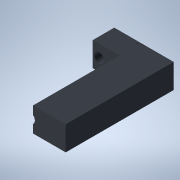
# Autodesk Inventor part: FGR AL-2-PGN-plus-P 160,PGN-plus-P 160-2-AS-P81110452001216049.51650000000000000000Aluminium6.5
Saved by Autodesk Inventor 2021 (Build 250183000, 183)
## iProperties
Created: 2025-07-30
Part Number: FGR AL-2-PGN-plus-P 160,PGN-plus-P 160-2-AS-P81110452001216049.51650000000000000000Aluminium6.5
Material: Generic
Catalog Web Link: www.cadenas.de
Description: FGR-Customizable gripper fingers
Vendor: SCHUNK
Document SubType Name: Modeling
Designer: psAdmin
Manufacturer: SCHUNK
Mass: 613.504 g
Surface Area: 597.818 cm^2
Volume: 613.504 cm^3
Density: 1 g/cm^3
Appearance: PSOLRGB-188-193-204
Category: PARTsolutions
Company: SCHUNK
Title: FGR AL-2-PGN-plus-P 160, 110452002
Author: Cadenas PARTsolutions
Comments: Customizable gripper fingers
PSOL_IDENT_0: {$CADENAS_DATA/23d-libs/schunk/greifsysteme/konfigurationen/system_baukasten/easy_finger/easy_finger
PSOL_IDENT_1: _0421.prj},471 {VTYP=3D},{NB=FGR AL-2-PGN-plus-P 160,PGN-plus-P 160-2-AS-P81110452001216049.51650000
PSOL_IDENT_2: 000000000000Aluminium6.5},{LINA=FGR AL-2-PGN-plus-P 160, 110452002},{NN=FGR},{DATE=13.11.2024 09:26:
PSOL_IDENT_3: 27},{GEOMDATE=20.06.2024 14:57:51},{VERSION=},{LINEID=10},{WBVAR=BR,BGVR,ASIS,SPANNKONT,CNSMAT,HUB,R
PSOL_IDENT_4: H,X,Y,Z,ABK,DWS,GFL,GFT,PP,PW,RA,EFO,FASE1,FL1,FASE2,FL2,FASE3,FW3,FL3,FASE4,FW4,FL4,WAERMEBE,BM},{W
PSOL_IDENT_5: BNUMERIC=HUB,RH,X,Y,Z,ABK,DWS,GFL,GFT,PP,PW,RA,EFO,FL1,FL2,FASE3,FW3,FL3,FW4,FL4,BM}  {NB=FGR AL-2-P
PSOL_IDENT_6: GN-plus-P 160,PGN-plus-P 160-2-AS-P81110452001216049.51650000000000000000Aluminium6.5},{LINA=FGR AL-
PSOL_IDENT_7: 2-PGN-plus-P 160, 110452002},{KT=DUMMY},{START=Geometriemodell 2},{VERSION=1},{VER=V1},{MATN=3786171
PSOL_IDENT_8: 200_fgr_gl_ia_v1},{XMLMATN=material|},{XMLMAT=AlZn55MgCu_EN-AW-7075_34365},{TYP=FGR AL-2-PGN-plus-P
PSOL_IDENT_9: 160},{TYPX=PGN-plus-P 160},{TYPXX=PGN-plus-P 160},{TYPXMAT=AL},{BR=PGN-plus-P},{BG=160.0},{BGVR=PGN-
PSOL_IDENT_10: plus-P 160-2-AS-P},{BGVRX='PGN-plus-P 40','PGN-plus-P 40','PGN-plus-P 40-SD','PGN-plus-P 40-SD','PGN
PSOL_IDENT_11: -plus-P 40-K','PGN-plus-P 40-K','PGN-plus-P 40-V','PGN-plus-P 40-V','PGN-plus-P 40-P','PGN-plus-P 40
PSOL_IDENT_12: -P','PGN-plus-P 40-AS','PGN-plus-P 40-AS','PGN-plus-P 40-AS-SD','PGN-plus-P 40-AS-SD','PGN-plus-P 40
PSOL_IDENT_13: -AS-K','PGN-plus-P 40-AS-K','PGN-plus-P 40-AS-V','PGN-plus-P 40-AS-V','PGN-plus-P 40-AS-P','PGN-plus
PSOL_IDENT_14: -P 40-AS-P','PGN-plus-P 40-IS','PGN-plus-P 40-IS','PGN-plus-P 40-IS-SD','PGN-plus-P 40-IS-SD','PGN-p
PSOL_IDENT_15: lus-P 40-IS-K','PGN-plus-P 40-IS-K','PGN-plus-P 40-IS-V','PGN-plus-P 40-IS-V','PGN-plus-P 50-1','PGN
PSOL_IDENT_16: -plus-P 50-1','PGN-plus-P 50-1-SD','PGN-plus-P 50-1-SD','PGN-plus-P 50-1-K','PGN-plus-P 50-1-K','PGN
PSOL_IDENT_17: -plus-P 50-1-V','PGN-plus-P 50-1-V','PGN-plus-P 50-1-P','PGN-plus-P 50-1-P','PGN-plus-P 50-2','PGN-p
PSOL_IDENT_18: lus-P 50-2','PGN-plus-P 50-2-SD','PGN-plus-P 50-2-SD','PGN-plus-P 50-2-K','PGN-plus-P 50-2-K','PGN-p
PSOL_IDENT_19: lus-P 50-2-V','PGN-plus-P 50-2-V','PGN-plus-P 50-2-P','PGN-plus-P 50-2-P','PGN-plus-P 50-1-AS','PGN-
PSOL_IDENT_20: plus-P 50-1-AS','PGN-plus-P 50-1-AS-SD','PGN-plus-P 50-1-AS-SD','PGN-plus-P 50-1-AS-K','PGN-plus-P 5
PSOL_IDENT_21: 0-1-AS-K','PGN-plus-P 50-1-AS-V','PGN-plus-P 50-1-AS-V','PGN-plus-P 50-1-AS-P','PGN-plus-P 50-1-AS-P'
PSOL_IDENT_22: ,'PGN-plus-P 50-2-AS','PGN-plus-P 50-2-AS','PGN-plus-P 50-2-AS-SD','PGN-plus-P 50-2-AS-SD','PGN-plus
PSOL_IDENT_23: -P 50-2-AS-K','PGN-plus-P 50-2-AS-K','PGN-plus-P 50-2-AS-V','PGN-plus-P 50-2-AS-V','PGN-plus-P 50-2-
PSOL_IDENT_24: AS-P','PGN-plus-P 50-2-AS-P','PGN-plus-P 50-1-IS','PGN-plus-P 50-1-IS','PGN-plus-P 50-1-IS-SD','PGN-
PSOL_IDENT_25: plus-P 50-1-IS-SD','PGN-plus-P 50-1-IS-K','PGN-plus-P 50-1-IS-K','PGN-plus-P 50-1-IS-V','PGN-plus-P
PSOL_IDENT_26: 50-1-IS-V','PGN-plus-P 50-2-IS','PGN-plus-P 50-2-IS','PGN-plus-P 50-2-IS-SD','PGN-plus-P 50-2-IS-SD'
PSOL_IDENT_27: ,'PGN-plus-P 50-2-IS-K','PGN-plus-P 50-2-IS-K','PGN-plus-P 50-2-IS-V','PGN-plus-P 50-2-IS-V','PGN-pl
PSOL_IDENT_28: us-P 64-1','PGN-plus-P 64-1','PGN-plus-P 64-1-SD','PGN-plus-P 64-1-SD','PGN-plus-P 64-1-K','PGN-plus
PSOL_IDENT_29: -P 64-1-K','PGN-plus-P 64-1-V','PGN-plus-P 64-1-V','PGN-plus-P 64-1-P','PGN-plus-P 64-1-P','PGN-plus
PSOL_IDENT_30: -P 64-2','PGN-plus-P 64-2','PGN-plus-P 64-2-SD','PGN-plus-P 64-2-SD','PGN-plus-P 64-2-K','PGN-plus-P
PSOL_IDENT_31: 64-2-K','PGN-plus-P 64-2-V','PGN-plus-P 64-2-V','PGN-plus-P 64-2-P','PGN-plus-P 64-2-P','PGN-plus-P
PSOL_IDENT_32: 64-1-AS','PGN-plus-P 64-1-AS','PGN-plus-P 64-1-AS-SD','PGN-plus-P 64-1-AS-SD','PGN-plus-P 64-1-AS-K'
PSOL_IDENT_33: ,'PGN-plus-P 64-1-AS-K','PGN-plus-P 64-1-AS-V','PGN-plus-P 64-1-AS-V','PGN-plus-P 64-1-AS-P','PGN-pl
PSOL_IDENT_34: us-P 64-1-AS-P','PGN-plus-P 64-2-AS','PGN-plus-P 64-2-AS','PGN-plus-P 64-1-IS','PGN-plus-P 64-1-IS','
PSOL_IDENT_35: PGN-plus-P 64-1-IS-SD','PGN-plus-P 64-1-IS-SD','PGN-plus-P 64-1-IS-K','PGN-plus-P 64-1-IS-K','PGN-pl
PSOL_IDENT_36: us-P 64-1-IS-V','PGN-plus-P 64-1-IS-V','PGN-plus-P 64-2-IS','PGN-plus-P 64-2-IS','PGN-plus-P 64-2-IS
PSOL_IDENT_37: -SD','PGN-plus-P 64-2-IS-SD','PGN-plus-P 64-2-IS-K','PGN-plus-P 64-2-IS-K','PGN-plus-P 64-2-V','PGN-
PSOL_IDENT_38: plus-P 64-2-V','PGN-plus-P 80-1','PGN-plus-P 80-1','PGN-plus-P 80-1-SD','PGN-plus-P 80-1-SD','PGN-pl
PSOL_IDENT_39: us-P 80-1-K','PGN-plus-P 80-1-K','PGN-plus-P 80-1-V','PGN-plus-P 80-1-V','PGN-plus-P 80-1-P','PGN-pl
PSOL_IDENT_40: us-P 80-1-P','PGN-plus-P 80-2','PGN-plus-P 80-2','PGN-plus-P 80-2-SD','PGN-plus-P 80-2-SD','PGN-plus
PSOL_IDENT_41: -P 80-2-K','PGN-plus-P 80-2-K','PGN-plus-P 80-2-V','PGN-plus-P 80-2-V','PGN-plus-P 80-2-P','PGN-plus
PSOL_IDENT_42: -P 80-2-P','PGN-plus-P 80-1-AS','PGN-plus-P 80-1-AS','PGN-plus-P 80-1-AS-SD','PGN-plus-P 80-1-AS-SD'
PSOL_IDENT_43: ,'PGN-plus-P 80-1-AS-K','PGN-plus-P 80-1-AS-K','PGN-plus-P 80-1-AS-V','PGN-plus-P 80-1-AS-V','PGN-pl
PSOL_IDENT_44: us-P 80-1-AS-P','PGN-plus-P 80-1-AS-P','PGN-plus-P 80-2-AS','PGN-plus-P 80-2-AS','PGN-plus-P 80-2-AS
PSOL_IDENT_45: -SD', 'PGN-plus-P 80-2-AS-SD','PGN-plus-P 80-2-AS-K','PGN-plus-P 80-2-AS-K','PGN-plus-P 80-2-AS-V','
PSOL_IDENT_46: PGN-plus-P 80-2-AS-V','PGN-plus-P 80-2-AS-P','PGN-plus-P 80-2-AS-P','PGN-plus-P 80-1-IS','PGN-plus-P
PSOL_IDENT_47: 80-1-IS','PGN-plus-P 80-1-IS-SD','PGN-plus-P 80-1-IS-SD','PGN-plus-P 80-1-IS-K','PGN-plus-P 80-1-IS
PSOL_IDENT_48: -K','PGN-plus-P 80-1-IS-V','PGN-plus-P 80-1-IS-V','PGN-plus-P 80-2-IS','PGN-plus-P 80-2-IS','PGN-plu
PSOL_IDENT_49: s-P 80-2-IS-SD','PGN-plus-P 80-2-IS-SD','PGN-plus-P 80-2-IS-K','PGN-plus-P 80-2-IS-K','PGN-plus-P 80
PSOL_IDENT_50: -2-IS-V','PGN-plus-P 80-2-IS-V','PGN-plus-P 100-1','PGN-plus-P 100-1','PGN-plus-P 100-1-SD','PGN-plu
PSOL_IDENT_51: s-P 100-1-SD','PGN-plus-P 100-1-K','PGN-plus-P 100-1-K','PGN-plus-P 100-1-V','PGN-plus-P 100-1-V','P
PSOL_IDENT_52: GN-plus-P 100-1-P','PGN-plus-P 100-1-P','PGN-plus-P 100-2','PGN-plus-P 100-2','PGN-plus-P 100-2-SD','
PSOL_IDENT_53: PGN-plus-P 100-2-SD','PGN-plus-P 100-2-K','PGN-plus-P 100-2-K','PGN-plus-P 100-2-V','PGN-plus-P 100-
PSOL_IDENT_54: 2-V','PGN-plus-P 100-2-P','PGN-plus-P 100-2-P','PGN-plus-P 100-1-AS','PGN-plus-P 100-1-AS','PGN-plus
PSOL_IDENT_55: -P 100-1-AS-SD','PGN-plus-P 100-1-AS-SD','PGN-plus-P 100-1-AS-K','PGN-plus-P 100-1-AS-K','PGN-plus-P
PSOL_IDENT_56: 100-1-AS-V','PGN-plus-P 100-1-AS-V','PGN-plus-P 100-1-AS-P','PGN-plus-P 100-1-AS-P','PGN-plus-P 100
PSOL_IDENT_57: -2-AS','PGN-plus-P 100-2-AS','PGN-plus-P 100-2-AS-SD','PGN-plus-P 100-2-AS-SD','PGN-plus-P 100-2-AS-
PSOL_IDENT_58: K','PGN-plus-P 100-2-AS-K','PGN-plus-P 100-2-AS-V','PGN-plus-P 100-2-AS-V','PGN-plus-P 100-2-AS-P','
PSOL_IDENT_59: PGN-plus-P 100-2-AS-P','PGN-plus-P 100-1-IS','PGN-plus-P 100-1-IS','PGN-plus-P 100-1-IS-SD','PGN-plu
PSOL_IDENT_60: s-P 100-1-IS-SD','PGN-plus-P 100-1-IS-K','PGN-plus-P 100-1-IS-K','PGN-plus-P 100-1-IS-V','PGN-plus-P
PSOL_IDENT_61: 100-1-IS-V','PGN-plus-P 100-2-IS','PGN-plus-P 100-2-IS','PGN-plus-P 100-2-IS-SD','PGN-plus-P 100-2-
PSOL_IDENT_62: IS-SD','PGN-plus-P 100-2-IS-K','PGN-plus-P 100-2-IS-K','PGN-plus-P 100-2-IS-V','PGN-plus-P 100-2-IS-
PSOL_IDENT_63: V','PGN-plus-P 125-1','PGN-plus-P 125-1','PGN-plus-P 125-1-SD','PGN-plus-P 125-1-SD','PGN-plus-P 125
PSOL_IDENT_64: -1-K','PGN-plus-P 125-1-K','PGN-plus-P 125-1-V','PGN-plus-P 125-1-V','PGN-plus-P 125-1-P','PGN-plus-
PSOL_IDENT_65: P 125-1-P','PGN-plus-P 125-2','PGN-plus-P 125-2','PGN-plus-P 125-2-SD','PGN-plus-P 125-2-SD','PGN-pl
PSOL_IDENT_66: us-P 125-2-K','PGN-plus-P 125-2-K','PGN-plus-P 125-2-V','PGN-plus-P 125-2-V','PGN-plus-P 125-2-P','P
PSOL_IDENT_67: GN-plus-P 125-2-P','PGN-plus-P 125-1-AS','PGN-plus-P 125-1-AS','PGN-plus-P 125-1-AS-SD','PGN-plus-P
PSOL_IDENT_68: 125-1-AS-SD','PGN-plus-P 125-1-AS-K','PGN-plus-P 125-1-AS-K','PGN-plus-P 125-1-AS-V','PGN-plus-P 125
PSOL_IDENT_69: -1-AS-V','PGN-plus-P 125-1-AS-P','PGN-plus-P 125-1-AS-P','PGN-plus-P 125-2-AS','PGN-plus-P 125-2-AS'
PSOL_IDENT_70: ,'PGN-plus-P 125-2-AS-SD','PGN-plus-P 125-2-AS-SD','PGN-plus-P 125-2-AS-K','PGN-plus-P 125-2-AS-K','
PSOL_IDENT_71: PGN-plus-P 125-2-AS-V','PGN-plus-P 125-2-AS-V','PGN-plus-P 125-2-AS-P','PGN-plus-P 125-2-AS-P','PGN-
PSOL_IDENT_72: plus-P 125-1-IS','PGN-plus-P 125-1-IS','PGN-plus-P 125-1-IS-SD','PGN-plus-P 125-1-IS-SD','PGN-plus-P
PSOL_IDENT_73: 125-1-IS-K','PGN-plus-P 125-1-IS-K','PGN-plus-P 125-1-IS-V','PGN-plus-P 125-1-IS-V','PGN-plus-P 125
PSOL_IDENT_74: -2-IS','PGN-plus-P 125-2-IS','PGN-plus-P 125-2-IS-SD','PGN-plus-P 125-2-IS-SD','PGN-plus-P 125-2-IS-
PSOL_IDENT_75: K','PGN-plus-P 125-2-IS-K','PGN-plus-P 125-2-IS-V','PGN-plus-P 125-2-IS-V','PGN-plus-P 160-1','PGN-p
PSOL_IDENT_76: lus-P 160-1','PGN-plus-P 160-1-SD','PGN-plus-P 160-1-SD','PGN-plus-P 160-1-K','PGN-plus-P 160-1-K','
PSOL_IDENT_77: PGN-plus-P 160-1-V','PGN-plus-P 160-1-V','PGN-plus-P 160-1-P','PGN-plus-P 160-1-P','PGN-plus-P 160-2'
PSOL_IDENT_78: ,'PGN-plus-P 160-2','PGN-plus-P 160-2-SD','PGN-plus-P 160-2-SD','PGN-plus-P 160-2-K','PGN-plus-P 160
PSOL_IDENT_79: -2-K','PGN-plus-P 160-2-V','PGN-plus-P 160-2-V','PGN-plus-P 160-2-P','PGN-plus-P 160-2-P','PGN-plus-
PSOL_IDENT_80: P 160-1-AS','PGN-plus-P 160-1-AS','PGN-plus-P 160-1-AS-SD','PGN-plus-P 160-1-AS-SD','PGN-plus-P 160-
PSOL_IDENT_81: 1-AS-K','PGN-plus-P 160-1-AS-K','PGN-plus-P 160-1-AS-V','PGN-plus-P 160-1-AS-V','PGN-plus-P 160-1-AS
PSOL_IDENT_82: -P','PGN-plus-P 160-1-AS-P','PGN-plus-P 160-2-AS','PGN-plus-P 160-2-AS','PGN-plus-P 160-2-AS-SD','PG
PSOL_IDENT_83: N-plus-P 160-2-AS-SD','PGN-plus-P 160-2-AS-K','PGN-plus-P 160-2-AS-K','PGN-plus-P 160-2-AS-V','PGN-p
PSOL_IDENT_84: lus-P 160-2-AS-V','PGN-plus-P 160-2-AS-P','PGN-plus-P 160-2-AS-P','PGN-plus-P 160-1-IS','PGN-plus-P
PSOL_IDENT_85: 160-1-IS','PGN-plus-P 160-1-IS-SD','PGN-plus-P 160-1-IS-SD','PGN-plus-P 160-1-IS-K','PGN-plus-P 160-
PSOL_IDENT_86: 1-IS-K','PGN-plus-P 160-1-IS-V','PGN-plus-P 160-1-IS-V','PGN-plus-P 160-2-IS','PGN-plus-P 160-2-IS','
PSOL_IDENT_87: PGN-plus-P 160-2-IS-SD','PGN-plus-P 160-2-IS-SD','PGN-plus-P 160-2-IS-K','PGN-plus-P 160-2-IS-K','PG
PSOL_IDENT_88: N-plus-P 160-2-IS-V','PGN-plus-P 160-2-IS-V','PGN-plus-P 200-1','PGN-plus-P 200-1','PGN-plus-P 200-1
PSOL_IDENT_89: -SD','PGN-plus-P 200-1-SD','PGN-plus-P 200-1-K','PGN-plus-P 200-1-K','PGN-plus-P 200-1-V','PGN-plus-
PSOL_IDENT_90: P 200-1-V','PGN-plus-P 200-1-P','PGN-plus-P 200-1-P','PGN-plus-P 200-2','PGN-plus-P 200-2','PGN-plus
PSOL_IDENT_91: -P 200-2-SD','PGN-plus-P 200-2-SD','PGN-plus-P 200-2-K','PGN-plus-P 200-2-K','PGN-plus-P 200-2-V','P
PSOL_IDENT_92: GN-plus-P 200-2-V','PGN-plus-P 200-2-P','PGN-plus-P 200-2-P','PGN-plus-P 200-1-AS','PGN-plus-P 200-1
PSOL_IDENT_93: -AS','PGN-plus-P 200-1-AS-SD','PGN-plus-P 200-1-AS-SD','PGN-plus-P 200-1-AS-K','PGN-plus-P 200-1-AS-
PSOL_IDENT_94: K','PGN-plus-P 200-1-AS-V','PGN-plus-P 200-1-AS-V','PGN-plus-P 200-1-AS-P','PGN-plus-P 200-1-AS-P','
PSOL_IDENT_95: PGN-plus-P 200-2-AS','PGN-plus-P 200-2-AS','PGN-plus-P 200-2-AS-SD','PGN-plus-P 200-2-AS-SD','PGN-pl
PSOL_IDENT_96: us-P 200-2-AS-K','PGN-plus-P 200-2-AS-K','PGN-plus-P 200-2-AS-V','PGN-plus-P 200-2-AS-V','PGN-plus-P
PSOL_IDENT_97: 200-2-AS-P','PGN-plus-P 200-2-AS-P','PGN-plus-P 200-1-IS','PGN-plus-P 200-1-IS','PGN-plus-P 200-1-I
PSOL_IDENT_98: S-SD','PGN-plus-P 200-1-IS-SD','PGN-plus-P 200-1-IS-K','PGN-plus-P 200-1-IS-K','PGN-plus-P 200-1-IS-
PSOL_IDENT_99: V','PGN-plus-P 200-1-IS-V','PGN-plus-P 200-2-IS','PGN-plus-P 200-2-IS','PGN-plus-P 200-2-IS-SD','PGN
PSOL_IDENT_100: -plus-P 200-2-IS-SD','PGN-plus-P 200-2-IS-K','PGN-plus-P 200-2-IS-K','PGN-plus-P 200-2-IS-V','PGN-pl
PSOL_IDENT_101: us-P 200-2-IS-V','PGN-plus-P 240-1','PGN-plus-P 240-1','PGN-plus-P 240-1-SD','PGN-plus-P 240-1-SD','
PSOL_IDENT_102: PGN-plus-P 240-1-K','PGN-plus-P 240-1-K','PGN-plus-P 240-1-V','PGN-plus-P 240-1-V','PGN-plus-P 240-1
PSOL_IDENT_103: -P','PGN-plus-P 240-1-P','PGN-plus-P 240-2','PGN-plus-P 240-2','PGN-plus-P 240-2-SD','PGN-plus-P 240
PSOL_IDENT_104: -2-SD','PGN-plus-P 240-2-K','PGN-plus-P 240-2-K','PGN-plus-P 240-2-V','PGN-plus-P 240-2-V','PGN-plus
PSOL_IDENT_105: -P 240-2-P','PGN-plus-P 240-2-P', 'PGN-plus-P 240-1-AS','PGN-plus-P 240-1-AS','PGN-plus-P 240-1-AS-S
PSOL_IDENT_106: D','PGN-plus-P 240-1-AS-SD','PGN-plus-P 240-1-AS-K','PGN-plus-P 240-1-AS-K','PGN-plus-P 240-1-AS-V','
PSOL_IDENT_107: PGN-plus-P 240-1-AS-V','PGN-plus-P 240-1-AS-P','PGN-plus-P 240-1-AS-P', 'PGN-plus-P 240-2-AS','PGN-p
PSOL_IDENT_108: lus-P 240-2-AS','PGN-plus-P 240-2-AS-SD','PGN-plus-P 240-2-AS-SD','PGN-plus-P 240-2-AS-K','PGN-plus-
PSOL_IDENT_109: P 240-2-AS-K','PGN-plus-P 240-2-AS-V','PGN-plus-P 240-2-AS-V','PGN-plus-P 240-2-AS-P','PGN-plus-P 24
PSOL_IDENT_110: 0-2-AS-P', 'PGN-plus-P 240-1-IS','PGN-plus-P 240-1-IS','PGN-plus-P 240-1-IS-SD','PGN-plus-P 240-1-IS
PSOL_IDENT_111: -SD','PGN-plus-P 240-1-IS-K','PGN-plus-P 240-1-IS-K','PGN-plus-P 240-1-IS-V','PGN-plus-P 240-1-IS-V'
PSOL_IDENT_112: , 'PGN-plus-P 240-2-IS','PGN-plus-P 240-2-IS','PGN-plus-P 240-2-IS-SD','PGN-plus-P 240-2-IS-SD','PGN
PSOL_IDENT_113: -plus-P 240-2-IS-K','PGN-plus-P 240-2-IS-K','PGN-plus-P 240-2-IS-V','PGN-plus-P 240-2-IS-V','PGN-plu
PSOL_IDENT_114: s-P 300-1','PGN-plus-P 300-1','PGN-plus-P 300-1-SD','PGN-plus-P 300-1-SD','PGN-plus-P 300-1-K','PGN-
PSOL_IDENT_115: plus-P 300-1-K','PGN-plus-P 300-1-V','PGN-plus-P 300-1-V','PGN-plus-P 300-1-P','PGN-plus-P 300-1-P','
PSOL_IDENT_116: PGN-plus-P 300-2','PGN-plus-P 300-2','PGN-plus-P 300-2-SD','PGN-plus-P 300-2-SD','PGN-plus-P 300-2-K'
PSOL_IDENT_117: ,'PGN-plus-P 300-2-K','PGN-plus-P 300-2-V','PGN-plus-P 300-2-V','PGN-plus-P 300-2-P','PGN-plus-P 300
PSOL_IDENT_118: -2-P', 'PGN-plus-P 300-1-AS','PGN-plus-P 300-1-AS','PGN-plus-P 300-1-AS-SD','PGN-plus-P 300-1-AS-SD'
PSOL_IDENT_119: ,'PGN-plus-P 300-1-AS-K','PGN-plus-P 300-1-AS-K','PGN-plus-P 300-1-AS-V','PGN-plus-P 300-1-AS-V','PG
PSOL_IDENT_120: N-plus-P 300-1-AS-P','PGN-plus-P 300-1-AS-P', 'PGN-plus-P 300-2-AS','PGN-plus-P 300-2-AS','PGN-plus-
PSOL_IDENT_121: P 300-2-AS-SD','PGN-plus-P 300-2-AS-SD','PGN-plus-P 300-2-AS-K','PGN-plus-P 300-2-AS-K','PGN-plus-P
PSOL_IDENT_122: 300-2-AS-V','PGN-plus-P 300-2-AS-V','PGN-plus-P 300-2-AS-P','PGN-plus-P 300-2-AS-P', 'PGN-plus-P 300
PSOL_IDENT_123: -1-IS','PGN-plus-P 300-1-IS','PGN-plus-P 300-1-IS-SD','PGN-plus-P 300-1-IS-SD','PGN-plus-P 300-1-IS-
PSOL_IDENT_124: K','PGN-plus-P 300-1-IS-K','PGN-plus-P 300-1-IS-V','PGN-plus-P 300-1-IS-V', 'PGN-plus-P 300-2-IS','P
PSOL_IDENT_125: GN-plus-P 300-2-IS','PGN-plus-P 300-2-IS-SD','PGN-plus-P 300-2-IS-SD','PGN-plus-P 300-2-IS-K','PGN-p
PSOL_IDENT_126: lus-P 300-2-IS-K','PGN-plus-P 300-2-IS-V','PGN-plus-P 300-2-IS-V','PGN-plus-P 380-1','PGN-plus-P 380
PSOL_IDENT_127: -1','PGN-plus-P 380-1-SD','PGN-plus-P 380-1-SD','PGN-plus-P 380-1-K','PGN-plus-P 380-1-K','PGN-plus-
PSOL_IDENT_128: P 380-1-V','PGN-plus-P 380-1-V','PGN-plus-P 380-1-P','PGN-plus-P 380-1-P','PGN-plus-P 380-2','PGN-pl
PSOL_IDENT_129: us-P 380-2','PGN-plus-P 380-2-SD','PGN-plus-P 380-2-SD','PGN-plus-P 380-2-K','PGN-plus-P 380-2-K','P
PSOL_IDENT_130: GN-plus-P 380-2-V','PGN-plus-P 380-2-V','PGN-plus-P 380-2-P','PGN-plus-P 380-2-P', 'PGN-plus-P 380-1
PSOL_IDENT_131: -AS','PGN-plus-P 380-1-AS','PGN-plus-P 380-1-AS-SD','PGN-plus-P 380-1-AS-SD','PGN-plus-P 380-1-AS-K'
PSOL_IDENT_132: ,'PGN-plus-P 380-1-AS-K','PGN-plus-P 380-1-AS-V','PGN-plus-P 380-1-AS-V','PGN-plus-P 380-1-AS-P','PG
PSOL_IDENT_133: N-plus-P 380-1-AS-P', 'PGN-plus-P 380-2-AS','PGN-plus-P 380-2-AS','PGN-plus-P 380-2-AS-SD','PGN-plus
PSOL_IDENT_134: -P 380-2-AS-SD','PGN-plus-P 380-2-AS-K','PGN-plus-P 380-2-AS-K','PGN-plus-P 380-2-AS-V','PGN-plus-P
PSOL_IDENT_135: 380-2-AS-V','PGN-plus-P 380-2-AS-P','PGN-plus-P 380-2-AS-P', 'PGN-plus-P 380-1-IS','PGN-plus-P 380-1
PSOL_IDENT_136: -IS','PGN-plus-P 380-1-IS-SD','PGN-plus-P 380-1-IS-SD','PGN-plus-P 380-1-IS-K','PGN-plus-P 380-1-IS-
PSOL_IDENT_137: K','PGN-plus-P 380-1-IS-V','PGN-plus-P 380-1-IS-V', 'PGN-plus-P 380-2-IS','PGN-plus-P 380-2-IS','PGN
PSOL_IDENT_138: -plus-P 380-2-IS-SD','PGN-plus-P 380-2-IS-SD','PGN-plus-P 380-2-IS-K','PGN-plus-P 380-2-IS-K','PGN-p
PSOL_IDENT_139: lus-P 380-2-IS-V','PGN-plus-P 380-2-IS-V'},{IDNR=1317660},{ASIS=1},{ASISX=<'1','Außengreifen','ausse
PSOL_IDENT_140: ngreifen.png'>,'2','Innnengreifen','innengreifen.png'},{ASISXX=AS},{SPANNKONT=2},{SPANNKONTX='1', 'G
PSOL_IDENT_141: erader Greiferfinger', 'startmodell_1.png', '2' , 'Greiferfinger mit nach innen abgesetzter Greifflä
PSOL_IDENT_142: che', 'startmodell_2.png', '3' , 'Greiferfinger mit nach außen abgesetzter Greiffläche', 'startmodel
PSOL_IDENT_143: l_3.png', '4' , 'Greiferfinger mit nach innen abgesetzter und abgerundeter Greiffläche', 'startmodel
PSOL_IDENT_144: l_4.png', '5' , 'Greiferfinger mit nach außen abgesetzter und abgerundeter Greiffläche', 'startmodel
PSOL_IDENT_145: l_5.png', '6' , 'Greiferfinger mit nach innen abgesetzter Greiffläche und vertikalem Prisma', 'start
PSOL_IDENT_146: modell_6.png','8' , 'Greiferfinger mit horizontalem Prisma', 'startmodell_8.png'},{CNSMAT=Aluminium}
PSOL_IDENT_147: ,{HUB=8.0},{HMAX=8.0},{RH=6.5},{HMAXX=8.0},{RHB=2.0},{AB=32.0},{GFM=38.50},{GFMAS=38.50},{GFMIS=70.5
PSOL_IDENT_148: 0},{X=110.0},{XMIN=56.0},{XMAX=113.0},{XTEST=[56:113/0.1]},{MAXX=113.0},{Y=45.0},{YMIN=27.0},{YMAX=6
PSOL_IDENT_149: 0.0},{MAXY=60.0},{Z=200.0},{ZMIN=32.0},{ZMAX=200.0},{ZMAXX=100.0},{MAXZ=200.0},{ABK=12.00},{ABKMIN=1
PSOL_IDENT_150: 2.00},{ABKMAX=37.50},{DWS=165.0},{DWSX=[68:222]},{DWSMIN=68.000},{DWSMAX=222.000},{DWSMAXX=111.0},{D
PSOL_IDENT_151: WSXX=1.000},{DWSZ=1.000},{DWS1V=70.0},{DWS1H=110.0},{DWS2V=134.0},{DWS2H=174.0},{DWSK=134.0},{GWI=1.
PSOL_IDENT_152: 0},{GFL=160.0},{GFLX=[1:169.4]},{GFLMIN=1.00},{GFLMAX=169.40},{GFT=49.50},{GFTX=[49.5:49.5/0.1]},{GF
PSOL_IDENT_153: TMIN=49.50},{GFTMINTH=-217577236067824.12},{GFTMAX=49.50},{GFT1V=2.00},{GFT1H=22.00},{GFT2V=34.00},{
PSOL_IDENT_154: GFT2H=54.00},{SKS=10.6},{PP=0.0},{PPX=[0]},{PPMIN=0.0},{PPMAX=0.0},{PUK=0.00},{PUKZ=88.50},{PUKX=0.0
PSOL_IDENT_155: 0},{PW=0.0},{PWX=[0]},{PWMIN=120},{PWMAX=120},{PWTH=120.0},{PWTHX=180.000},{ALPHA=0.000},{RA=0.0},{R
PSOL_IDENT_156: AX=[0]},{RAMIN=1},{RAMAX=44},{EFO=0.0},{EFOX=[0]},{EFOMAX=0.10},{FASE1=0},{FASE1X='0','ohne Fase 1','
PSOL_IDENT_157: kein_bild.png','1','mit Fase 1','fase_1.png'},{FW1=0.0},{FL1=0.0},{FL1MIN=0.0},{FL1MAX=0.0},{FASE2=0
PSOL_IDENT_158: },{FASE2X='0','ohne Fase 2','kein_bild.png','1','mit Fase 2','fase_2.png'},{FW2=0.0},{FL2=0.0},{FL2M
PSOL_IDENT_159: IN=0.0},{FL2MAX=0.00},{FASE3=0},{FW3=0.0},{FW3MIN=0.0},{FW3MAX=0.0},{FL3=0.0},{FL3MIN=0.0},{FL3MAX=0
PSOL_IDENT_160: .00},{FASE4=0},{FASE4X='0','ohne Fase 4','kein_bild.png','1','mit Fase 4','fase_4_glatt.png'},{FW4=0
PSOL_IDENT_161: .0},{FW4MIN=0.0},{FW4MAX=0.0},{FL4=0.0},{FL4MIN=0.0},{FL4MAX=0.00},{ROHX=2.683},{ROH=1.457},{ZULFM=3
PSOL_IDENT_162: .800},{VALFM=true},{VOL=537767.200},{VFASE1=0.00},{VFASE2=0.00},{VFASE3=0.00},{VFASE4=0.00},{GFTXX=2
PSOL_IDENT_163: .00},{STX1=20.00},{STX2=20.00},{EST=17.0},{ZD=14.0},{ZT=4.0},{DB=11.0},{SD=18.0},{ST=20.0},{RI=8.2},
PSOL_IDENT_164: {L=6.5},{LX=-31},{L1=1.000},{L1X=-0.000},{L2=1.000},{LA=82.500},{GANS=M10},{PBO=11.0},{DPB=11.00},{R
PSOL_IDENT_165: PO=3},{AQB=2.75},{SCHT=0.75},{SCHL=17.40},{SCHH=6.40},{SCHP=5.00},{TYPALU=3.00},{SCHGD=10.0},{SCHGL=
PSOL_IDENT_166: 35.0},{LZ=5 Werktage},{VK=272.00},{VKB=226.11},{VKZ=33.92},{VKX=11.31},{VKP=0.00},{ZX=200.00},{ZXX=1
PSOL_IDENT_167: 00.00},{XX=113.00},{XXX=56.50},{SPERR=0.00},{WC=3786171200_fgr_gl_ia_v1.prt},{MN=3786171200_FGR_GL_I
PSOL_IDENT_168: A_V1},{XMLX=dim|15},{XMLY=dim|14},{XMLZ=dim|13},{XMLAB=dim|35},{XMLABK=dim|71},{XMLGFL=dim|70},{XMLG
PSOL_IDENT_169: FT=dim|68},{XMLFL1=dim|188},{XMLFL2=dim|151},{XMLFL3=dim|272},{XMLFW3=dim|274},{XMLFL4=dim|212},{XML
PSOL_IDENT_170: FW4=dim|211},{XMLRA=},{XMLRI=},{XMLPW=},{XMLDWS=para|DWS},{XMLGFM=para|GFM},{XMLRH=},{XMLEFO=},{XMLP
PSOL_IDENT_171: P=},{XMLASIS=para|ASIS},{XMLVER=para|1|VER},{ANZ=2},{SG3D=8.0},{WAERMEBEX='',''},{WAERMEBE=},{SAPWAE
PSOL_IDENT_172: RMEBE=10},{DICHTE=2.71},{SAPLZ=5},{VKW=0.00},{BM=2}
NB: FGR AL-2-PGN-plus-P 160,PGN-plus-P 160-2-AS-P81110452001216049.51650000000000000000Aluminium6.5
NN: FGR
NT: Customizable gripper fingers
NBSYN: $TYP.,$BGVR.$HUB.$ASIS.$X.$Y.$Z.$ABK.$GFL.$GFT.$DWS.$PP.$PW.$RA.$EFO.$FASE1.$FW1.$FL1.$FASE2.$FW2.$FL2.$FASE3.$FW3.$FL3.$FASE4.$FW4.$FL4.$CNSMAT.$RH.
LINA: FGR AL-2-PGN-plus-P 160, 110452002
CATALOG: SCHUNK
VER: V1
XMLMATN: material|
TYP: FGR AL-2-PGN-plus-P 160
BR: PGN-plus-P
BGVR: PGN-plus-P 160-2-AS-P
ASIS: O.D. gripping
SPANNKONT: Gripper finger with inwardly stepped gripping surface
CNSMAT: Aluminium AlZnMgCu1,5
HUB: 8
RH: 6.5
AB: 32
GFM: 38.5
X: 110
Y: 45
Z: 200
ABK: 12
DWS: 165
GFL: 160
GFT: 49.5
PP: 0
PW: 0
RA: 0
EFO: 0
FASE1: without chamfer 1
FW1: 0
FL1: 0
FASE2: without chamfer 2
FW2: 0
FL2: 0
FASE3: without chamfer 3
FW3: 0
FL3: 0
FASE4: without chamfer 4
FW4: 0
FL4: 0
LZ: 5 working days
VK: 272
XMLDWS: para|DWS
XMLGFM: para|GFM
XMLASIS: para|ASIS
XMLVER: para|1|VER
BM: 2
SUPPLIER: SCHUNK
ARTICLENO: FGR AL-2-PGN-plus-P 160,PGN-plus-P 160-2-AS-P81110452001216049.51650000000000000000Aluminium6.5
BOMINFO: FGR AL-2-PGN-plus-P 160, 110452002
CREATOR: CADENAS GmbH
Autodesk Inventor part; units mm, degrees
sketch "Sketch_1" plane through (0, 0, 0) normal (0, 0, 1) x (1, 0, 0)
  line L0 (-12, -22.5) -> (98, -22.5)
  line L1 (98, -22.5) -> (98, 22.5)
  line L2 (98, 22.5) -> (-12, 22.5)
  line L3 (-12, 22.5) -> (-12, -22.5)
  constraints: 8 end point
extrude "Extrusion1" add sketch "Sketch_1" along normal blind 200
sketch "Sketch_2" plane through (0, 0, 0) normal (0, 1, 0) x (-1, 0, 0)
  line L0 (0, 200) -> (0, 0)
  line L1 (0, 0) -> (-7, 0)
  line L2 (-7, 0) -> (-7, 4)
  line L3 (-7, 4) -> (-5.5, 4)
  line L4 (-5.5, 4) -> (-5.5, 20)
  line L5 (-5.5, 20) -> (-9, 20)
  line L6 (-9, 20) -> (-9, 200)
  line L7 (-9, 200) -> (0, 200)
  line L8 (0, 200) -> (0, 0)
  constraints: 18 end point
revolve "Revolution1" cut sketch "Sketch_2" angle 360 about axis through (0, 0, 200) along (0, 0, 1)
pattern_linear "Rectangular Pattern1" count 2 spacing 32 along (1, 0, 0) of "Revolution1"
sketch "Sketch_8" plane through (0, 0, 200) normal (0, 0, 1) x (1, 0, 0)
  line L0 (-12, -22.5) -> (37.5, -22.5)
  line L1 (37.5, -22.5) -> (37.5, 22.5)
  line L2 (37.5, 22.5) -> (-12, 22.5)
  line L3 (-12, 22.5) -> (-12, -22.5)
  constraints: 8 end point
extrude "Extrusion2" cut sketch "Sketch_8" against normal blind 160
sketch "Sketch_17" plane through (0, 22.5, 0) normal (0, 1, 0) x (1, 0, 0)
  arc A0 (37.5, -1.8) -> (37.5, -8.2) centre (37.5, -5) ccw
  line L0 (37.5, -8.2) -> (48.5, -8.2)
  arc A1 (48.5, -8.2) -> (48.5, -1.8) centre (48.5, -5) ccw
  line L1 (48.5, -1.8) -> (37.5, -1.8)
  constraints: 4 end point, 4 point on circle, 2 centre point
extrude "Extrusion3" cut sketch "Sketch_17" against normal blind 0.75
ref_plane "BEF_2_XY" through (32, 0, 0) normal (0, 0, 1) x (1, 0, 0)
ref_plane "BEF_2_YZ" through (32, 0, 0) normal (1, 0, 0) x (0, 1, 0)
ref_plane "BEF_2_ZX" through (32, 0, 0) normal (0, 1, 0) x (0, 0, 1)
ref_plane "IP_ALU_XY" through (43, 21.75, 5) normal (0, -1, 0) x (1, 0, 0)
ref_plane "IP_ALU_YZ" through (43, 21.75, 5) normal (1, 0, 0) x (0, 0, 1)
ref_plane "IP_ALU_ZX" through (43, 21.75, 5) normal (0, 0, 1) x (0, -1, 0)
ref_plane "IP_ALU_3_7_XY" through (44, 21.75, 5) normal (0, -1, 0) x (1, 0, 0)
ref_plane "IP_ALU_3_7_YZ" through (44, 21.75, 5) normal (1, 0, 0) x (0, 0, 1)
ref_plane "IP_ALU_3_7_ZX" through (44, 21.75, 5) normal (0, 0, 1) x (0, -1, 0)
ref_plane "IP_ALU_5_XY" through (44, 21.75, 5) normal (0, -1, 0) x (1, 0, 0)
ref_plane "IP_ALU_5_YZ" through (44, 21.75, 5) normal (1, 0, 0) x (0, 0, 1)
ref_plane "IP_ALU_5_ZX" through (44, 21.75, 5) normal (0, 0, 1) x (0, -1, 0)
ref_plane "IP_GR_XY" through (0, 0, 0) normal (0, 0, 1) x (1, 0, 0)
ref_plane "IP_GR_YZ" through (0, 0, 0) normal (1, 0, 0) x (0, 1, 0)
ref_plane "IP_GR_ZX" through (0, 0, 0) normal (0, 1, 0) x (0, 0, 1)
ref_plane "IP_SCH_1_XY" through (0, 0, 20) normal (0, 0, 1) x (1, 0, 0)
ref_plane "IP_SCH_1_YZ" through (0, 0, 20) normal (1, 0, 0) x (0, 1, 0)
ref_plane "IP_SCH_1_ZX" through (0, 0, 20) normal (0, 1, 0) x (0, 0, 1)
ref_plane "IP_SCH_2_XY" through (32, 0, 20) normal (0, 0, 1) x (1, 0, 0)
ref_plane "IP_SCH_2_YZ" through (32, 0, 20) normal (1, 0, 0) x (0, 1, 0)
ref_plane "IP_SCH_2_ZX" through (32, 0, 20) normal (0, 1, 0) x (0, 0, 1)
body "Solid1"
